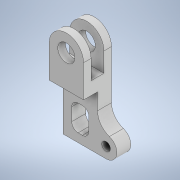
# Autodesk Inventor part: 2번부품
Saved by Autodesk Inventor 2022 (Build 260153000, 153)
## iProperties
Created: 2021-09-05
Part Number: 2번부품
Material: 일반
Document SubType Name: Modeling
Designer: 서울공업고등학교
Density: 1 g/cm^3
Appearance: 기본값
Author: 서울공업고등학교
Autodesk Inventor part; units mm, degrees
ref_plane "YZ Plane" through (0, 0, 0) normal (1, 0, 0) x (0, 1, 0)
ref_plane "XZ Plane" through (0, 0, 0) normal (0, 1, 0) x (-1, 0, 0)
ref_plane "XY Plane" through (0, 0, 0) normal (0, 0, 1) x (1, 0, 0)
sketch "스케치1" plane through (0, 0, 0) normal (0, 0, 1) x (1, 0, 0)
  line L0 (0, 0) -> (16, 0)
  line L1 (16, 48) -> (0, 48)
  line L2 (0, 48) -> (0, 0)
  line L3 (0, 0) -> (20, 0)
  line L4 (0, 0) -> (20, 0) construction
  circle A0 centre (20, 5) radius 2
  line L5 (20, 10) -> (16, 10)
  circle A1 centre (20, 5) radius 5
  line L6 (16, 48) -> (16, 10)
  circle A2 centre (8, 40) radius 4
  line L7 (4, 16) -> (12, 16)
  line L8 (12, 16) -> (12, 4)
  line L9 (12, 4) -> (4, 4)
  line L10 (4, 4) -> (4, 16)
  line L11 (0, 25) -> (16, 25)
  dimension "d0" = 16
  dimension "d4" = 48
  dimension "d5" = 20
  dimension "d8" = 4
  dimension "d9" = 10
  dimension "d10" = 8
  dimension "d11" = 40
  dimension "d12" = 8
  dimension "d13" = 12
  dimension "d14" = 4
  dimension "d15" = 4
  dimension "d16" = 8
  dimension "d17" = 25
  constraints: 24 end point, 5 horizontal, 3 centre point, 3 parallel, 2 perpendicular, 2 point on line, 2 tangent, 1 coincident, 1 collinear, 1 vertical, 1 vertical alignment
  measures "d0" distance of L1.end L1.start
  measures "d4" distance of L1.end L0.start
  measures "d5" distance of L0.start L3.end
  measures "d8" diameter of A0
  measures "d9" diameter of A1
  measures "d10" diameter of A2
  measures "d11" distance from line of L0 A2.centre
  measures "d12" distance between parallel lines of L8 L10
  measures "d13" distance between parallel lines of L9 L7
  measures "d14" distance between parallel lines of L3 L9
  measures "d15" distance between parallel lines of L10 L2
  measures "d16" distance from line of A2.centre L2
  measures "d17" distance between parallel lines of L0 L11
extrude "돌출1" add sketch "스케치1" against normal blind 6.5 contours L2 L11 L6 L5 A1 L3 L0 | A1
extrude "돌출2" add sketch "스케치1" along normal mid plane 13 contours L2 L1 L6 L11
fillet "모깎기1" radius 8 2 edges at (16, 48, 0) (0, 48, 0)
fillet "모깎기2" radius 3 4 edges at (4, 16, -3.25) (12, 16, -3.25) (12, 4, -3.25) (4, 4, -3.25)
fillet "모깎기3" radius 8 1 edges at (16, 10, -3.25)
sketch "스케치2" plane through (0, 0, 0) normal (0, 0, 1) x (1, 0, 0)
  line L0 (-9.7469, 60.6249) -> (29.3105, 60.6249)
  line L1 (29.3105, 60.6249) -> (29.3105, 31)
  line L2 (29.3105, 31) -> (-9.7469, 31)
  line L3 (-9.7469, 31) -> (-9.7469, 60.6249)
  point P0 (0, 0)
  dimension "d25" = 31
  constraints: 8 end point, 2 parallel, 1 horizontal, 1 perpendicular
  measures "d25" distance from line of point (0, 0) L2
extrude "돌출3" cut sketch "스케치2" along normal mid plane 6
